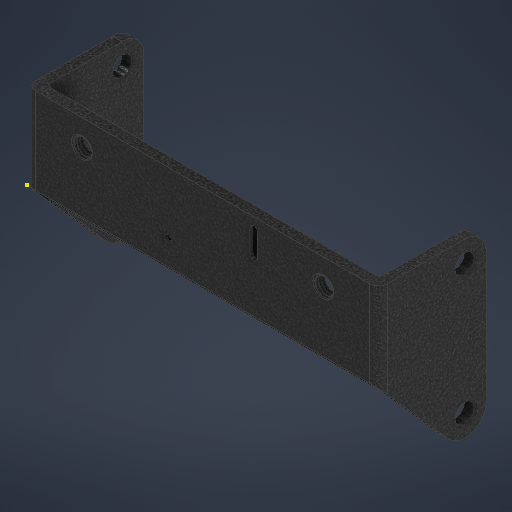
# Autodesk Inventor part: LaserBeslag
Saved by Autodesk Inventor 2026.2 (Build 302298010, 298A)
## iProperties
Created: 2026-04-22
Part Number: LaserBeslag
Material: PET Plastic
Document SubType Name: Modeling
Designer: frede
Density: 1.541 g/cm^3
Appearance: Black Cast
Author: frede
Autodesk Inventor part; units mm, degrees
ref_plane "YZ Plane" through (0, 0, 0) normal (1, 0, 0) x (0, 1, 0)
ref_plane "XZ Plane" through (0, 0, 0) normal (0, 1, 0) x (-1, 0, 0)
ref_plane "XY Plane" through (0, 0, 0) normal (0, 0, 1) x (1, 0, 0)
sketch "Sketch1" plane through (0, 0, 0) normal (1, 0, 0) x (0, 1, 0)
  circle A0 centre (-37.5, 0) radius 5.5
  circle A1 centre (37.5, 0) radius 5.5
  line L0 (-50, 50) -> (50, 50)
  line L1 (50, 50) -> (50, -12.5)
  line L2 (50, -12.5) -> (-50, -12.5)
  line L3 (-50, -12.5) -> (-50, 50)
  point P0 (0, 0)
  point P1 (42.6235, -2)
  point P2 (32.3765, -2)
  point P3 (-32.3765, -2)
  point P4 (-42.6235, -2)
  dimension "d0" = 11
  dimension "d1" = 11
  dimension "d2" = 100
  dimension "d3" = 62.5
  dimension "d42" = 12.5
  dimension "d43" = 12.5
  dimension "d44" = 12.5
  constraints: 8 end point, 2 centre point, 2 parallel, 1 horizontal, 1 perpendicular
  measures "d0" diameter of A0
  measures "d1" diameter of A1
  measures "d2" distance of L1.end L2.end
  measures "d3" distance of L0.end L1.end
  measures "d42" distance from line of L2 A0.centre
  measures "d43" distance from line of L3 A0.centre
  measures "d44" distance from line of L1 A1.centre
extrude "Extrusion1" add sketch "Sketch1" along normal blind 204
sketch "Sketch2" plane through (0, -50, -12.5) normal (0, -1, 0) x (1, 0, 0)
  line L0 (204, 0) -> (204, 62.5) projected
  line L1 (0, 0) -> (204, 0)
  line L2 (204, 0) -> (204, 62.5)
  line L3 (204, 62.5) -> (0, 62.5)
  line L4 (0, 62.5) -> (0, 0)
  line L5 (5.5, 0) -> (198.5, 0)
  line L6 (198.5, 0) -> (198.5, 56.5)
  line L7 (198.5, 56.5) -> (5.5, 56.5)
  line L8 (5.5, 56.5) -> (5.5, 0)
  point P0 (0, 12.5)
  point P1 (198.5, 0)
  dimension "d6" = 204
  dimension "d7" = 193
  dimension "d9" = 5.5
  dimension "d100" = 6
  constraints: 16 end point, 4 parallel, 2 horizontal, 2 perpendicular, 1 point on line
  measures "d6" distance between parallel lines of L0 L4
  measures "d7" distance of L7.end L6.end
  measures "d9" distance between parallel lines of L4 L8
  measures "d100" distance between parallel lines of L3 L7
extrude "Extrusion2" cut sketch "Sketch2" against normal up to surface (100 mm away) contours L1 L8 L7 L6
fillet "Fillet1" radius 12.5 4 edges at (201.25, 50, -12.5) (201.25, -50, -12.5) (2.75, 50, -12.5) (2.75, -50, -12.5)
fillet "Fillet2" radius 2 2 edges at (198.5, 0, 44) (5.5, 0, 44)
fillet "Fillet3" radius 5 2 edges at (204, 0, 50) (0, 0, 50)
sketch "Sketch4" plane through (196.5, -50, 44) normal (0, 0, -1) x (-1, 0, 0)
  line L0 (0, 100) -> (189, 100) projected
  line L1 (58.5, 100) -> (118.5, 100)
  line L2 (118.5, 100) -> (118.5, 58)
  line L3 (118.5, 58) -> (58.5, 58)
  line L4 (58.5, 58) -> (58.5, 100)
  arc A0 (60.9, 80) -> (68.9, 80) centre (64.9, 80) ccw
  circle A1 centre (114.9, 64) radius 4
  line L5 (-7.5, 12.5) -> (-7.5, 87.5) projected
  line L6 (94.5, 58) -> (94.5, 100)
  line L7 (196.5, 12.5) -> (196.5, 87.5) projected
  arc A2 (62.6, 80) -> (67.2, 80) centre (64.9, 80) ccw
  line L8 (64.9, 80) -> (64.9, 93.4)
  arc A3 (68.9, 93.4) -> (60.9, 93.4) centre (64.9, 93.4) ccw
  line L9 (60.9, 93.4) -> (60.9, 80)
  line L10 (68.9, 93.4) -> (68.9, 80)
  arc A4 (67.2, 93.4) -> (62.6, 93.4) centre (64.9, 93.4) ccw
  line L11 (62.6, 93.4) -> (62.6, 80)
  line L12 (67.2, 93.4) -> (67.2, 80)
  point P0 (196.5, 50)
  dimension "d15" = 60
  dimension "d16" = 42
  dimension "d17" = 8
  dimension "d19" = 6.4
  dimension "d20" = 8
  dimension "d22" = 6
  dimension "d24" = 36
  dimension "d25" = 102
  dimension "d26" = 204
  dimension "d34" = 16
  dimension "d36" = 50
  dimension "d47" = 4.6
  dimension "d48" = 13.4
  dimension "d49" = 8
  dimension "d50" = 4.6
  constraints: 20 end point, 8 point on circle, 6 tangent, 5 centre point, 3 coincident, 3 point on line, 3 vertical, 2 parallel, 2 perpendicular, 1 horizontal
  measures "d15" distance of L2.end L3.end
  measures "d16" distance of L1.end L2.end
  measures "d17" diameter of A0
  measures "d19" distance from line of L4 A0.centre
  measures "d20" diameter of A1
  measures "d22" distance from line of L3 A1.centre
  measures "d24" distance between parallel lines of L4 L6
  measures "d25" distance between parallel lines of L6 L5
  measures "d26" distance between parallel lines of L7 L5
  measures "d34" vertical distance of A1.centre A0.centre
  measures "d36" horizontal distance of A1.centre A0.centre
  measures "d47" diameter of A2
  measures "d48" distance of L8.start L8.end
  measures "d49" diameter of A3
  measures "d50" diameter of A4
extrude "Extrusion3" cut sketch "Sketch4" against normal blind 4 contours A1 L2 | L2 A1 | L9 A3 L10 A0 | L11 A4 L12 A2
sketch "Sketch5" plane through (131.6, 30, 48) normal (0, 0, -1) x (-1, 0, 0)
  arc A0 (-4, 0) -> (4, 0) centre (0, 0) ccw projected
  circle A1 centre (50, -16) radius 4 projected
  arc A2 (-2.125, 0) -> (2.125, 0) centre (0, 0) ccw
  circle A3 centre (50, -16) radius 2.125
  arc A4 (4, 13.4) -> (-4, 13.4) centre (0, 13.4) ccw projected
  arc A5 (2.125, 13.4) -> (-2.125, 13.4) centre (0, 13.4) ccw
  line L0 (-2.125, 0) -> (-2.125, 13.4)
  line L1 (2.125, 13.4) -> (2.125, 0)
  point P0 (131.6, -30)
  dimension "d29" = 4.25
  dimension "d30" = 4.25
  dimension "d51" = 4.25
  constraints: 5 coincident, 4 end point, 4 point on circle, 3 centre point, 3 tangent
  measures "d29" diameter of A2
  measures "d30" diameter of A3
  measures "d51" diameter of A5
extrude "Extrusion4" cut sketch "Sketch5" against normal blind 6 contours L0 A5 L1 A2 | A3
sketch "Sketch6" plane through (204, 0, 0) normal (1, 0, 0) x (0, 0, -1)
  line L0 (-50, -50) -> (-12.5, -50)
  line L1 (-12.5, -39) -> (-12.5, -36)
  line L2 (-42, -50) -> (0, -50) projected
  line L3 (-1.5, -50) -> (0, -50)
  circle A0 centre (0, -37.5) radius 5.5 projected
  line L4 (12.5, -37.5) -> (12.5, 37.5) projected
  arc A1 (-9.3485, -45.798) -> (12.5, -37.5) centre (0, -37.5) ccw
  line L5 (-50, 50) -> (-50, -50) projected
  line L6 (-50, 0) -> (-9.3485, -45.798)
  line L7 (-50, 0) -> (-50, -50)
  point P0 (0, 0)
  dimension "d39" = 14
  constraints: 10 end point, 3 point on circle, 3 point on line, 2 collinear, 1 centre point, 1 coincident, 1 horizontal, 1 midpoint, 1 tangent, 1 vertical
  measures "d39" distance of L0.end L1.end
extrude "Extrusion5" cut sketch "Sketch6" against normal up to surface (204 mm away) contours L5 L6 A1 L2 L0
sketch "Sketch7" plane through (5, 50, 50) normal (0, 0, 1) x (1, 0, 0)
  point P0 (-5, -50)
sketch "Sketch8" plane through (5, 50, 50) normal (0, 0, 1) x (1, 0, 0)
  circle A0 centre (167, -15) radius 6
  circle A1 centre (27, -15) radius 6
  line L0 (0, -50) -> (0, 0) projected
  line L1 (194, 0) -> (194, -50) projected
  line L2 (0, 0) -> (194, 0) projected
  point P0 (-5, -50)
  point P1 (0, -53.9706)
  point P2 (194, -53.9706)
  point P3 (0, -100)
  point P4 (194, -100)
  dimension "d52" = 12
  dimension "d53" = 12
  dimension "d54" = 140
  dimension "d55" = 194
  dimension "d56" = 27
  dimension "d57" = 15
  constraints: 2 centre point
  measures "d52" diameter of A0
  measures "d53" diameter of A1
  measures "d54" distance of A1.centre A0.centre
  measures "d55" distance between parallel lines of L0 L1
  measures "d56" distance from line of A0.centre L1
  measures "d57" distance from line of A1.centre L2
extrude "Extrusion6" cut sketch "Sketch8" against normal up to surface (6 mm away)
thread "Thread3" size "M12x1.75" class "6H" standard "ISO Metric profile" full length
thread "Thread4" size "M12x1.75" class "6H" standard "ISO Metric profile" full length
sketch "Sketch14" plane through (172, 35, 44) normal (1, 0, 0) x (0, 1, 0)
  line L0 (6, 0) -> (6, 6)
  line L1 (6, 6) -> (4.7024, 6)
  line L2 (4.7024, 6) -> (4.7024, 0)
  line L3 (4.7024, 0) -> (6, 0)
  line L4 (0, -69) -> (0, 18.5) projected
  constraints: 8 end point
revolve "Revolution3" add sketch "Sketch14" angle 360 about axis through (172, 35, 44) along (0, 0, 1) separate body
sketch "Sketch13" plane through (172, 41, 44) normal (-1, 0, 0) x (0, 0, 1)
  line L0 (-1.0209, -0.0887) -> (-0.8751, -0.0887) construction
  line L1 (0.1457, -1.2092) -> (-0.0001, -1.4894) construction
  line L2 (-1.7501, -1.4894) -> (-1.8959, -1.2092) construction
  line L3 (-0.7293, -0.0887) -> (-0.8751, 0.1915) construction
  line L4 (-0.8751, 0.1915) -> (-1.0209, -0.0887) construction
  line L5 (-1.7501, -1.4894) -> (-1.6043, -1.2092) construction
  line L6 (-0.7293, -0.0887) -> (-0.1459, -1.2092)
  line L7 (-1.8959, -1.2092) -> (-1.6043, -1.2092) construction
  arc A0 (-1.8959, -1.2092) -> (-1.7501, -1.2977) centre (-1.7501, -1.1333) ccw construction
  line L8 (0.1457, -1.2092) -> (-0.1459, -1.2092) construction
  line L9 (-1.7501, -1.4894) -> (-1.7501, -1.2092) construction
  line L10 (-0.0001, -1.4894) -> (-0.0001, -1.2092) construction
  line L11 (-0.8751, 0.1915) -> (-0.8751, -0.0002) construction
  line L12 (-1.7501, -1.2977) -> (-0.0001, -1.2977)
  arc A1 (-1.7501, -1.2977) -> (-1.6043, -1.2092) centre (-1.7501, -1.1333) ccw
  line L13 (-0.1459, -1.2092) -> (-0.0001, -1.4894) construction
  line L14 (-1.6043, -1.2092) -> (-1.0209, -0.0887)
  line L15 (-0.0001, -0.0002) -> (-0.0001, 0.0177)
  line L16 (-0.0001, 0.0177) -> (-0.0001, -0.0002)
  line L17 (-0.0001, -0.0002) -> (0.0334, -0.0002)
  arc A2 (-0.1459, -1.2092) -> (-0.0001, -1.2977) centre (-0.0001, -1.1333) ccw
  arc A3 (-0.0001, -1.2977) -> (0.1457, -1.2092) centre (-0.0001, -1.1333) ccw construction
  arc A4 (-0.8751, -0.0002) -> (-1.0209, -0.0887) centre (-0.8751, -0.1646) ccw
  arc A5 (-0.7293, -0.0887) -> (-0.8751, -0.0002) centre (-0.8751, -0.1646) ccw
  line L18 (-0.8751, -0.0002) -> (-0.8751, -0.0887) construction
  line L19 (-0.8751, -0.0887) -> (-0.7293, -0.0887) construction
  dimension "d105" = 55
  dimension "d106" = 0.2802
  dimension "d107" = 0.2802
  dimension "Sketch13_ThreadOffset" = 0
  dimension "Sketch13_MajorRadius" = 1.2976
  dimension "d110" = 1.75
  dimension "Sketch13_MinorRadius" = 0
  constraints: 40 end point, 12 point on circle, 10 parallel, 8 tangent, 6 centre point, 6 collinear, 2 midpoint, 2 point on line, 1 horizontal, 1 perpendicular, 3 other
  measures "d105" angle of L6 L14
  measures "d106" distance of L3.end L0.end
  measures "d107" distance of L1.end L10.end
  measures "Sketch13_ThreadOffset" distance between parallel lines of L15 L10
  measures "Sketch13_MajorRadius" distance from line of L12 L15.start
  measures "d110" distance from line of L1.end L9
  measures "Sketch13_MinorRadius" distance edge to line of A5 L17
coil "Coil3" sketch "Sketch13" operation cut axis through (172, 35, 44) along (0, 0, 1) pitch 1.785 turns 5.322129 hand right bodies 2
sketch "Sketch16" plane through (32, 35, 44) normal (1, 0, 0) x (0, 1, 0)
  line L0 (6, 0) -> (6, 6)
  line L1 (6, 6) -> (4.7024, 6)
  line L2 (4.7024, 6) -> (4.7024, 0)
  line L3 (4.7024, 0) -> (6, 0)
  line L4 (0, -69.1167) -> (0, 19.2) projected
  constraints: 8 end point
revolve "Revolution4" add sketch "Sketch16" angle 360 about axis through (32, 35, 44) along (0, 0, 1) separate body
sketch "Sketch15" plane through (32, 41, 44) normal (-1, 0, 0) x (0, 0, 1)
  line L0 (-1.0209, -0.0887) -> (-0.8751, -0.0887) construction
  line L1 (0.1457, -1.2092) -> (-0.0001, -1.4894) construction
  line L2 (-1.7501, -1.4894) -> (-1.8959, -1.2092) construction
  line L3 (-0.7293, -0.0887) -> (-0.8751, 0.1915) construction
  line L4 (-0.8751, 0.1915) -> (-1.0209, -0.0887) construction
  line L5 (-1.7501, -1.4894) -> (-1.6043, -1.2092) construction
  line L6 (-0.7293, -0.0887) -> (-0.1459, -1.2092)
  line L7 (-1.8959, -1.2092) -> (-1.6043, -1.2092) construction
  arc A0 (-1.8959, -1.2092) -> (-1.7501, -1.2977) centre (-1.7501, -1.1333) ccw construction
  line L8 (0.1457, -1.2092) -> (-0.1459, -1.2092) construction
  line L9 (-1.7501, -1.4894) -> (-1.7501, -1.2092) construction
  line L10 (-0.0001, -1.4894) -> (-0.0001, -1.2092) construction
  line L11 (-0.8751, 0.1915) -> (-0.8751, -0.0002) construction
  line L12 (-1.7501, -1.2977) -> (-0.0001, -1.2977)
  arc A1 (-1.7501, -1.2977) -> (-1.6043, -1.2092) centre (-1.7501, -1.1333) ccw
  line L13 (-0.1459, -1.2092) -> (-0.0001, -1.4894) construction
  line L14 (-1.6043, -1.2092) -> (-1.0209, -0.0887)
  line L15 (-0.0001, -0.0002) -> (-0.0001, 0.0177)
  line L16 (-0.0001, 0.0177) -> (-0.0001, -0.0002)
  line L17 (-0.0001, -0.0002) -> (0.0334, -0.0002)
  arc A2 (-0.1459, -1.2092) -> (-0.0001, -1.2977) centre (-0.0001, -1.1333) ccw
  arc A3 (-0.0001, -1.2977) -> (0.1457, -1.2092) centre (-0.0001, -1.1333) ccw construction
  arc A4 (-0.8751, -0.0002) -> (-1.0209, -0.0887) centre (-0.8751, -0.1646) ccw
  arc A5 (-0.7293, -0.0887) -> (-0.8751, -0.0002) centre (-0.8751, -0.1646) ccw
  line L18 (-0.8751, -0.0002) -> (-0.8751, -0.0887) construction
  line L19 (-0.8751, -0.0887) -> (-0.7293, -0.0887) construction
  dimension "d123" = 55
  dimension "d124" = 0.2802
  dimension "d125" = 0.2802
  dimension "Sketch15_ThreadOffset" = 0
  dimension "Sketch15_MajorRadius" = 1.2976
  dimension "d128" = 1.75
  dimension "Sketch15_MinorRadius" = 0
  constraints: 40 end point, 12 point on circle, 10 parallel, 8 tangent, 6 centre point, 6 collinear, 2 midpoint, 2 point on line, 1 horizontal, 1 perpendicular, 3 other
  measures "d123" angle of L6 L14
  measures "d124" distance of L3.end L0.end
  measures "d125" distance of L1.end L10.end
  measures "Sketch15_ThreadOffset" distance between parallel lines of L15 L10
  measures "Sketch15_MajorRadius" distance from line of L12 L15.start
  measures "d128" distance from line of L1.end L9
  measures "Sketch15_MinorRadius" distance edge to line of A5 L17
coil "Coil4" sketch "Sketch15" operation cut axis through (32, 35, 44) along (0, 0, 1) pitch 1.785 turns 5.322129 hand right bodies 3
equation "\"d9\" = -0.5 * d7 + 0.5 * d6"
equation "\"d25\" = 0.5 * d26"
equation "\"d50\" = d47"
equation "\"d56\" = -0.5 * d54 + 0.5 * d55"
equation "\"d105\" = d112"
equation "\"d106\" = 0.160083 * Sketch13_Pitch"
equation "\"d107\" = 0.160083 * Sketch13_Pitch"
equation "\"d110\" = Sketch13_Pitch"
equation "\"d123\" = d130"
equation "\"d124\" = 0.160083 * Sketch15_Pitch"
equation "\"d125\" = 0.160083 * Sketch15_Pitch"
equation "\"d128\" = Sketch15_Pitch"
equation "\"d71\" = 55deg"
equation "\"Sketch9_Pitch\" = 1.75"
equation "\"d89\" = 55deg"
equation "\"Sketch11_Pitch\" = 1.75"
equation "\"d112\" = 55deg"
equation "\"Sketch13_Pitch\" = 1.75"
equation "\"d130\" = 55deg"
equation "\"Sketch15_Pitch\" = 1.75"
body "Solid1"
body "Solid4"
body "Solid5"
